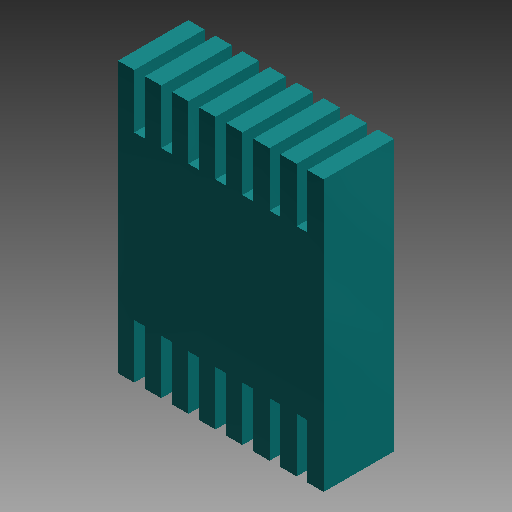
# Autodesk Inventor part: ADUM7441
Saved by Autodesk Inventor 2018.2 (Build 222227000, 227)
## iProperties
Part Number: ADUM7441
Material: Generic
Document SubType Name: Modeling
Designer: autocad
Appearance: QSOP16, ADUM7441
Author: autocad
Autodesk Inventor part; units mm, degrees
ref_plane "YZ Plane" through (0, 0, 0) normal (1, 0, 0) x (0, 1, 0)
ref_plane "XZ Plane" through (0, 0, 0) normal (0, 1, 0) x (-1, 0, 0)
ref_plane "XY Plane" through (0, 0, 0) normal (0, 0, 1) x (1, 0, 0)
sketch "QSOP16, ADUM7441_151" plane through (0, 0, 0) normal (0, 0, 1) x (1, 0, 0)
  line L0 (-2.032, 3.175) -> (-2.032, 1.905)
  line L1 (-2.032, 1.905) -> (-1.778, 1.905)
  line L2 (-1.778, 1.905) -> (-1.778, 3.175)
  line L3 (-1.778, 3.175) -> (-1.397, 3.175)
  line L4 (-1.397, 3.175) -> (-1.397, 1.905)
  line L5 (-1.397, 1.905) -> (-1.143, 1.905)
  line L6 (-1.143, 1.905) -> (-1.143, 3.175)
  line L7 (-1.143, 3.175) -> (-0.762, 3.175)
  line L8 (-0.762, 3.175) -> (-0.762, 1.905)
  line L9 (-0.762, 1.905) -> (-0.508, 1.905)
  line L10 (-0.508, 1.905) -> (-0.508, 3.175)
  line L11 (-0.508, 3.175) -> (-0.127, 3.175)
  line L12 (-0.127, 3.175) -> (-0.127, 1.905)
  line L13 (-0.127, 1.905) -> (0.127, 1.905)
  line L14 (0.127, 1.905) -> (0.127, 3.175)
  line L15 (0.127, 3.175) -> (0.508, 3.175)
  line L16 (0.508, 3.175) -> (0.508, 1.905)
  line L17 (0.508, 1.905) -> (0.762, 1.905)
  line L18 (0.762, 1.905) -> (0.762, 3.175)
  line L19 (0.762, 3.175) -> (1.143, 3.175)
  line L20 (1.143, 3.175) -> (1.143, 1.905)
  line L21 (1.143, 1.905) -> (1.397, 1.905)
  line L22 (1.397, 1.905) -> (1.397, 3.175)
  line L23 (1.397, 3.175) -> (1.778, 3.175)
  line L24 (1.778, 3.175) -> (1.778, 1.905)
  line L25 (1.778, 1.905) -> (2.032, 1.905)
  line L26 (2.032, 1.905) -> (2.032, 3.175)
  line L27 (2.032, 3.175) -> (2.413, 3.175)
  line L28 (2.413, 3.175) -> (2.413, -3.175)
  line L29 (2.413, -3.175) -> (2.032, -3.175)
  line L30 (2.032, -3.175) -> (2.032, -1.905)
  line L31 (2.032, -1.905) -> (1.778, -1.905)
  line L32 (1.778, -1.905) -> (1.778, -3.175)
  line L33 (1.778, -3.175) -> (1.397, -3.175)
  line L34 (1.397, -3.175) -> (1.397, -1.905)
  line L35 (1.397, -1.905) -> (1.143, -1.905)
  line L36 (1.143, -1.905) -> (1.143, -3.175)
  line L37 (1.143, -3.175) -> (0.762, -3.175)
  line L38 (0.762, -3.175) -> (0.762, -1.905)
  line L39 (0.762, -1.905) -> (0.508, -1.905)
  line L40 (0.508, -1.905) -> (0.508, -3.175)
  line L41 (0.508, -3.175) -> (0.127, -3.175)
  line L42 (0.127, -3.175) -> (0.127, -1.905)
  line L43 (0.127, -1.905) -> (-0.127, -1.905)
  line L44 (-0.127, -1.905) -> (-0.127, -3.175)
  line L45 (-0.127, -3.175) -> (-0.508, -3.175)
  line L46 (-0.508, -3.175) -> (-0.508, -1.905)
  line L47 (-0.508, -1.905) -> (-0.762, -1.905)
  line L48 (-0.762, -1.905) -> (-0.762, -3.175)
  line L49 (-0.762, -3.175) -> (-1.143, -3.175)
  line L50 (-1.143, -3.175) -> (-1.143, -1.905)
  line L51 (-1.143, -1.905) -> (-1.397, -1.905)
  line L52 (-1.397, -1.905) -> (-1.397, -3.175)
  line L53 (-1.397, -3.175) -> (-1.778, -3.175)
  line L54 (-1.778, -3.175) -> (-1.778, -1.905)
  line L55 (-1.778, -1.905) -> (-2.032, -1.905)
  line L56 (-2.032, -1.905) -> (-2.032, -3.175)
  line L57 (-2.032, -3.175) -> (-2.413, -3.175)
  line L58 (-2.413, -3.175) -> (-2.413, 3.175)
  line L59 (-2.413, 3.175) -> (-2.032, 3.175)
  constraints: 120 end point
extrude "Extrusion1" add sketch "QSOP16, ADUM7441_151" along normal blind 1.65
body "Solid1"
